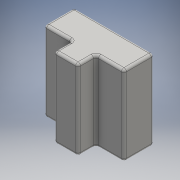
# Autodesk Inventor part: Kameratalpv3
Saved by Autodesk Inventor 2016 (Build 200138000, 138)
## iProperties
Created: 2018-03-31
Part Number: Kameratalpv3
Material: Generic
Document SubType Name: Modeling
Designer: bogna
Density: 1 g/cm^3
Appearance: Default
Author: bogna
Autodesk Inventor part; units mm, degrees
ref_plane "YZ Plane" through (0, 0, 0) normal (1, 0, 0) x (0, 1, 0)
ref_plane "XZ Plane" through (0, 0, 0) normal (0, 1, 0) x (-1, 0, 0)
ref_plane "XY Plane" through (0, 0, 0) normal (0, 0, 1) x (1, 0, 0)
sketch "Sketch1" plane through (0, 0, 0) normal (0, 0, 1) x (1, 0, 0)
  line L0 (-11.2, 0) -> (11.2, 0) projected
  line L1 (0, -11.52) -> (0, 1.92) projected
  line L2 (-8, 0) -> (8, 0)
  line L3 (8, -6) -> (2.4, -6)
  line L4 (2.4, -6) -> (2.4, -9.6)
  line L5 (2.4, -9.6) -> (-2.4, -9.6)
  line L6 (-2.4, -9.6) -> (-2.4, -6)
  line L7 (-2.4, -6) -> (-8, -6)
  line L8 (-8, -6) -> (-8, 0)
  line L9 (8, 0) -> (8, -6)
  point P0 (0, 0)
  dimension "d0" = 4.8
  dimension "d1" = 3.6
  dimension "d2" = 6
  dimension "d3" = 16
  constraints: 16 end point, 4 perpendicular, 4 point on line, 1 horizontal, 1 vertical, 2 other
  measures "d0" distance of L4.end L5.end
  measures "d1" distance of L3.end L4.end
  measures "d2" distance of L2.end L3.start
  measures "d3" distance between parallel lines of L9 L8
extrude "Extrusion1" add sketch "Sketch1" along normal mid plane 16
fillet "Fillet1" radius 0.5 8 edges at (8, -6, 0) (2.4, -6, 0) (2.4, -9.6, 0) (-2.4, -9.6, 0) (-8, -6, 0) (-2.4, -6, 0) (-8, 0, 0) (8, 0, 0)
sketch "Sketch2" plane through (0, 0, 0) normal (0, 0, 1) x (1, 0, 0)
  arc A0 (-4.6915, 0) -> (0, -3.1) centre (0, 2) ccw
  line L0 (7.5, 0) -> (-7.5, 0) construction
  line L1 (-4.6915, 0) -> (0, 0)
  line L2 (0, -3.1) -> (0, 0)
  line L3 (-4.6915, 0) -> (0, 0)
  line L4 (0, -4.966) -> (0, 3.161) projected
  dimension "d7" = 10.2
  dimension "d8" = 2
  constraints: 6 end point, 2 collinear, 2 point on circle, 1 centre point, 1 perpendicular, 1 point on line
  measures "d7" diameter of A0
  measures "d8" distance from line of L0 A0.centre
revolve "Revolution1" cut sketch "Sketch2" angle 360 about axis through (0, -10, 0) along (0, 1, 0)
fillet "Fillet2" radius 0.5 32 edges at (-7.8536, -0.1464, 8) (-8, -3, 8) (-7.8536, -5.8536, 8) (-5.2, -6, 8) (-2.5464, -6.1464, 8) (-2.4, -7.8, 8) (-2.2536, -9.4536, 8) (0, -9.6, 8) (2.2536, -9.4536, 8) (2.4, -7.8, 8) (2.5464, -6.1464, 8) (5.2, -6, 8) (7.8536, -5.8536, 8) (8, -3, 8) (7.8536, -0.1464, 8) (0, 0, 8) (7.8536, -0.1464, -8) (8, -3, -8) (7.8536, -5.8536, -8) (5.2, -6, -8) (2.5464, -6.1464, -8) (2.4, -7.8, -8) (2.2536, -9.4536, -8) (0, -9.6, -8) (-2.2536, -9.4536, -8) (-2.4, -7.8, -8) (-2.5464, -6.1464, -8) (-5.2, -6, -8) (-7.8536, -5.8536, -8) (-8, -3, -8) (-7.8536, -0.1464, -8) (0, 0, -8)
body "Solid1"
